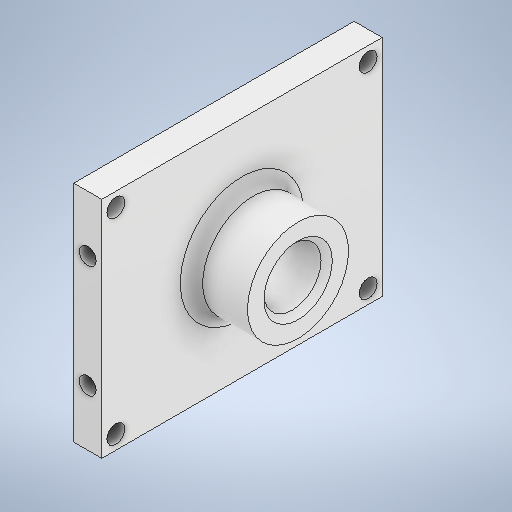
# Autodesk Inventor part: Handle_Front_End
Saved by Autodesk Inventor 2026.2 (Build 302298010, 298A)
## iProperties
Created: 2026-04-30
Part Number: Handle_Front_End
Material: ABS Plastic
Document SubType Name: Modeling
Designer: piete
Density: 1.06 g/cm^3
Appearance: Smooth - White
Author: piete
Autodesk Inventor part; units mm, degrees
ref_plane "YZ Plane" through (0, 0, 0) normal (1, 0, 0) x (0, 1, 0)
ref_plane "XZ Plane" through (0, 0, 0) normal (0, 1, 0) x (-1, 0, 0)
ref_plane "XY Plane" through (0, 0, 0) normal (0, 0, 1) x (1, 0, 0)
sketch "Sketch1" plane through (0, 0, 0) normal (1, 0, 0) x (0, 1, 0)
  line L0 (20, 25) -> (-20, 25)
  line L1 (-20, 25) -> (-20, -25)
  line L2 (-20, -25) -> (20, -25)
  line L3 (20, -25) -> (20, 25)
  point P0 (0, 0)
  dimension "d0" = 40
  dimension "d1" = 50
  dimension "d2" = 20
  dimension "d3" = 25
  constraints: 8 end point, 2 parallel, 1 horizontal, 1 perpendicular
  measures "d0" distance of L2.end L1.end
  measures "d1" distance of L1.end L0.end
  measures "d2" distance from line of point (0, 0) L3
  measures "d3" distance from line of L2 point (0, 0)
extrude "Extrusion1" add sketch "Sketch1" along normal blind 5
sketch "Sketch2" plane through (5, 0, 0) normal (1, 0, 0) x (0, 0, -1)
  circle A0 centre (0, 0) radius 5.1
  dimension "d6" = 10.2
  constraints: 1 centre point, 1 coincident
  measures "d6" diameter of A0
extrude "Extrusion2" cut sketch "Sketch2" against normal through all
sketch "Sketch3" plane through (5, 0, 0) normal (1, 0, 0) x (0, 0, -1)
  circle A0 centre (0, 0) radius 5.1
  circle A1 centre (0, 0) radius 9
  dimension "d9" = 10.2
  dimension "d10" = 18
  constraints: 2 centre point, 2 coincident
  measures "d9" diameter of A0
  measures "d10" diameter of A1
extrude "Extrusion3" add sketch "Sketch3" along normal blind 10
chamfer "Chamfer1" distance 1 angle 45 1 edges at (15, 0, 5.1)
fillet "Fillet1" radius 2 1 edges at (5, 0, 9)
sketch "Sketch4" plane through (5, 0, 0) normal (1, 0, 0) x (0, 0, -1)
  circle A0 centre (-22.5, 17.5) radius 1.6
  circle A1 centre (22.5, 17.5) radius 1.6
  circle A2 centre (22.5, -17.5) radius 1.6
  circle A3 centre (-22.5, -17.5) radius 1.6
  line L0 (-25, 20) -> (-25, -20) projected
  line L1 (25, 20) -> (-25, 20) projected
  line L2 (25, -20) -> (25, 20) projected
  line L3 (-25, -20) -> (25, -20) projected
  point P0 (0, 0)
  dimension "d17" = 3.2
  dimension "d18" = 3.2
  dimension "d19" = 3.2
  dimension "d20" = 3.2
  dimension "d21" = 2.5
  dimension "d22" = 2.5
  dimension "d23" = 2.5
  dimension "d24" = 2.5
  dimension "d25" = 2.5
  dimension "d26" = 2.5
  dimension "d27" = 2.5
  dimension "d28" = 2.5
  constraints: 4 centre point
  measures "d17" diameter of A0
  measures "d18" diameter of A1
  measures "d19" diameter of A2
  measures "d20" diameter of A3
  measures "d21" distance from line of L0 A0.centre
  measures "d22" distance from line of L1 A1.centre
  measures "d23" distance from line of L2 A2.centre
  measures "d24" distance from line of L0 A3.centre
  measures "d25" distance from line of L3 A3.centre
  measures "d26" distance from line of L3 A2.centre
  measures "d27" distance from line of L2 A1.centre
  measures "d28" distance from line of L1 A0.centre
extrude "Extrusion4" cut sketch "Sketch4" against normal through all contours A0 | A1 | A2 | A3
sketch "Sketch5" plane through (0, -20, 25) normal (0, 0, 1) x (1, 0, 0)
  circle A0 centre (2.5, 30) radius 1.5
  line L0 (0, 40) -> (0, 0) projected
  circle A1 centre (2.5, 10) radius 1.5
  point P0 (0, 20)
  point P1 (0, 20)
  point P2 (0, 20)
  dimension "d31" = 3
  dimension "d32" = 2.5
  dimension "d33" = 10
  dimension "d34" = 3
  dimension "d35" = 2.5
  dimension "d36" = 10
  constraints: 2 centre point, 2 midpoint
  measures "d31" diameter of A0
  measures "d32" distance from line of L0 A0.centre
  measures "d33" vertical distance of point (0, 20) A0.centre
  measures "d34" diameter of A1
  measures "d35" distance from line of L0 A1.centre
  measures "d36" vertical distance of point (0, 20) A1.centre
extrude "Extrusion5" cut sketch "Sketch5" against normal blind 5
mirror "Mirror1" about plane through (0, 0, 0) normal (0, 0, 1) of "Extrusion5"
equation "\"d2\" = 0.5 * d0"
equation "\"d3\" = 0.5 * d1"
body "Solid1"
